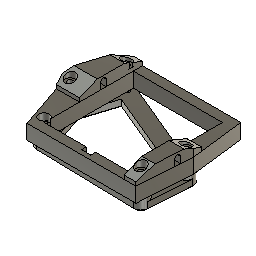
TF4060 rev 5 Heatsink holder (Autodesk Fusion 360 design; units mm, degrees)
Autodesk Fusion 360 part; units mm, degrees
(part 1 of 2)
sketch "68060 socket" plane through (0, 0, 0) normal (0, 0, 1) x (1, 0, 0)
  circle A0 centre (21.59, 21.59) radius 0.4
  circle A1 centre (19.05, 21.59) radius 0.4
  circle A2 centre (16.51, 21.59) radius 0.4
  circle A3 centre (13.97, 21.59) radius 0.4
  circle A4 centre (11.43, 21.59) radius 0.4
  circle A5 centre (8.89, 21.59) radius 0.4
  circle A6 centre (6.35, 21.59) radius 0.4
  circle A7 centre (3.81, 21.59) radius 0.4
  circle A8 centre (1.27, 21.59) radius 0.4
  circle A9 centre (-1.27, 21.59) radius 0.4
  circle A10 centre (-3.81, 21.59) radius 0.4
  circle A11 centre (-6.35, 21.59) radius 0.4
  circle A12 centre (-8.89, 21.59) radius 0.4
  circle A13 centre (-11.43, 21.59) radius 0.4
  circle A14 centre (-13.97, 21.59) radius 0.4
  circle A15 centre (-16.51, 21.59) radius 0.4
  circle A16 centre (-19.05, 21.59) radius 0.4
  circle A17 centre (21.59, 19.05) radius 0.4
  circle A18 centre (21.59, 16.51) radius 0.4
  circle A19 centre (21.59, 13.97) radius 0.4
  circle A20 centre (21.59, 11.43) radius 0.4
  circle A21 centre (21.59, 8.89) radius 0.4
  circle A22 centre (21.59, 6.35) radius 0.4
  circle A23 centre (21.59, 3.81) radius 0.4
  circle A24 centre (21.59, 1.27) radius 0.4
  circle A25 centre (21.59, -1.27) radius 0.4
  circle A26 centre (21.59, -3.81) radius 0.4
  circle A27 centre (21.59, -6.35) radius 0.4
  circle A28 centre (21.59, -8.89) radius 0.4
  circle A29 centre (21.59, -11.43) radius 0.4
  circle A30 centre (21.59, -13.97) radius 0.4
  circle A31 centre (21.59, -16.51) radius 0.4
  circle A32 centre (21.59, -19.05) radius 0.4
  circle A33 centre (21.59, -21.59) radius 0.4
  circle A34 centre (19.05, 19.05) radius 0.4
  circle A35 centre (19.05, 16.51) radius 0.4
  circle A36 centre (19.05, 13.97) radius 0.4
  circle A37 centre (16.51, 19.05) radius 0.4
  circle A38 centre (16.51, 16.51) radius 0.4
  circle A39 centre (16.51, 13.97) radius 0.4
  circle A40 centre (13.97, 19.05) radius 0.4
  circle A41 centre (13.97, 16.51) radius 0.4
  circle A42 centre (13.97, 13.97) radius 0.4
  circle A43 centre (11.43, 19.05) radius 0.4
  circle A44 centre (11.43, 16.51) radius 0.4
  circle A45 centre (11.43, 13.97) radius 0.4
  circle A46 centre (8.89, 19.05) radius 0.4
  circle A47 centre (8.89, 16.51) radius 0.4
  circle A48 centre (8.89, 13.97) radius 0.4
  circle A49 centre (6.35, 19.05) radius 0.4
  circle A50 centre (6.35, 16.51) radius 0.4
  circle A51 centre (6.35, 13.97) radius 0.4
  circle A52 centre (3.81, 19.05) radius 0.4
  circle A53 centre (3.81, 16.51) radius 0.4
  circle A54 centre (3.81, 13.97) radius 0.4
  circle A55 centre (1.27, 19.05) radius 0.4
  circle A56 centre (1.27, 16.51) radius 0.4
  circle A57 centre (1.27, 13.97) radius 0.4
  circle A58 centre (-1.27, 19.05) radius 0.4
  circle A59 centre (-1.27, 16.51) radius 0.4
  circle A60 centre (-1.27, 13.97) radius 0.4
  circle A61 centre (-3.81, 19.05) radius 0.4
  circle A62 centre (-3.81, 16.51) radius 0.4
  circle A63 centre (-3.81, 13.97) radius 0.4
  circle A64 centre (-6.35, 19.05) radius 0.4
  circle A65 centre (-6.35, 16.51) radius 0.4
  circle A66 centre (-6.35, 13.97) radius 0.4
  circle A67 centre (-8.89, 19.05) radius 0.4
  circle A68 centre (-8.89, 16.51) radius 0.4
  circle A69 centre (-8.89, 13.97) radius 0.4
  circle A70 centre (-11.43, 19.05) radius 0.4
  circle A71 centre (-11.43, 16.51) radius 0.4
  circle A72 centre (-11.43, 13.97) radius 0.4
  circle A73 centre (-13.97, 19.05) radius 0.4
  circle A74 centre (-13.97, 16.51) radius 0.4
  circle A75 centre (-13.97, 13.97) radius 0.4
  circle A76 centre (-16.51, 19.05) radius 0.4
  circle A77 centre (-16.51, 16.51) radius 0.4
  circle A78 centre (-16.51, 13.97) radius 0.4
  circle A79 centre (-19.05, 19.05) radius 0.4
  circle A80 centre (-19.05, 16.51) radius 0.4
  circle A81 centre (-19.05, 13.97) radius 0.4
  circle A82 centre (-21.59, 19.05) radius 0.4
  circle A83 centre (-21.59, 16.51) radius 0.4
  circle A84 centre (-21.59, 13.97) radius 0.4
  circle A85 centre (19.05, -21.59) radius 0.4
  circle A86 centre (19.05, -19.05) radius 0.4
  circle A87 centre (19.05, -16.51) radius 0.4
  circle A88 centre (19.05, -13.97) radius 0.4
  circle A89 centre (16.51, -21.59) radius 0.4
  circle A90 centre (16.51, -19.05) radius 0.4
  circle A91 centre (16.51, -16.51) radius 0.4
  circle A92 centre (16.51, -13.97) radius 0.4
  circle A93 centre (13.97, -21.59) radius 0.4
  circle A94 centre (13.97, -19.05) radius 0.4
  circle A95 centre (13.97, -16.51) radius 0.4
  circle A96 centre (13.97, -13.97) radius 0.4
  circle A97 centre (11.43, -21.59) radius 0.4
  circle A98 centre (11.43, -19.05) radius 0.4
  circle A99 centre (11.43, -16.51) radius 0.4
  circle A100 centre (11.43, -13.97) radius 0.4
  circle A101 centre (8.89, -21.59) radius 0.4
  circle A102 centre (8.89, -19.05) radius 0.4
  circle A103 centre (8.89, -16.51) radius 0.4
  circle A104 centre (8.89, -13.97) radius 0.4
  circle A105 centre (6.35, -21.59) radius 0.4
  circle A106 centre (6.35, -19.05) radius 0.4
  circle A107 centre (6.35, -16.51) radius 0.4
  circle A108 centre (6.35, -13.97) radius 0.4
  circle A109 centre (3.81, -21.59) radius 0.4
  circle A110 centre (3.81, -19.05) radius 0.4
  circle A111 centre (3.81, -16.51) radius 0.4
  circle A112 centre (3.81, -13.97) radius 0.4
  circle A113 centre (1.27, -21.59) radius 0.4
  circle A114 centre (1.27, -19.05) radius 0.4
  circle A115 centre (1.27, -16.51) radius 0.4
  circle A116 centre (1.27, -13.97) radius 0.4
  circle A117 centre (-1.27, -21.59) radius 0.4
  circle A118 centre (-1.27, -19.05) radius 0.4
  circle A119 centre (-1.27, -16.51) radius 0.4
  circle A120 centre (-1.27, -13.97) radius 0.4
  circle A121 centre (-3.81, -21.59) radius 0.4
  circle A122 centre (-3.81, -19.05) radius 0.4
  circle A123 centre (-3.81, -16.51) radius 0.4
  circle A124 centre (-3.81, -13.97) radius 0.4
  circle A125 centre (-6.35, -21.59) radius 0.4
  circle A126 centre (-6.35, -19.05) radius 0.4
  circle A127 centre (-6.35, -16.51) radius 0.4
  circle A128 centre (-6.35, -13.97) radius 0.4
  circle A129 centre (-8.89, -21.59) radius 0.4
  circle A130 centre (-8.89, -19.05) radius 0.4
  circle A131 centre (-8.89, -16.51) radius 0.4
  circle A132 centre (-8.89, -13.97) radius 0.4
  circle A133 centre (-11.43, -21.59) radius 0.4
  circle A134 centre (-11.43, -19.05) radius 0.4
  circle A135 centre (-11.43, -16.51) radius 0.4
  circle A136 centre (-11.43, -13.97) radius 0.4
  circle A137 centre (-13.97, -21.59) radius 0.4
  circle A138 centre (-13.97, -19.05) radius 0.4
  circle A139 centre (-13.97, -16.51) radius 0.4
  circle A140 centre (-13.97, -13.97) radius 0.4
  circle A141 centre (-16.51, -21.59) radius 0.4
  circle A142 centre (-16.51, -19.05) radius 0.4
  circle A143 centre (-16.51, -16.51) radius 0.4
  circle A144 centre (-16.51, -13.97) radius 0.4
  circle A145 centre (-19.05, -21.59) radius 0.4
  circle A146 centre (-19.05, -19.05) radius 0.4
  circle A147 centre (-19.05, -16.51) radius 0.4
  circle A148 centre (-19.05, -13.97) radius 0.4
  circle A149 centre (-21.59, -21.59) radius 0.4
  circle A150 centre (-21.59, -19.05) radius 0.4
  circle A151 centre (-21.59, -16.51) radius 0.4
  circle A152 centre (-21.59, -13.97) radius 0.4
  circle A153 centre (19.05, -11.43) radius 0.4
  circle A154 centre (16.51, -11.43) radius 0.4
  circle A155 centre (13.97, -11.43) radius 0.4
  circle A156 centre (-13.97, -11.43) radius 0.4
  circle A157 centre (-16.51, -11.43) radius 0.4
  circle A158 centre (-19.05, -11.43) radius 0.4
  circle A159 centre (-21.59, -11.43) radius 0.4
  circle A160 centre (19.05, -8.89) radius 0.4
  circle A161 centre (16.51, -8.89) radius 0.4
  circle A162 centre (13.97, -8.89) radius 0.4
  circle A163 centre (-13.97, -8.89) radius 0.4
  circle A164 centre (-16.51, -8.89) radius 0.4
  circle A165 centre (-19.05, -8.89) radius 0.4
  circle A166 centre (-21.59, -8.89) radius 0.4
  circle A167 centre (19.05, -6.35) radius 0.4
  circle A168 centre (16.51, -6.35) radius 0.4
  circle A169 centre (13.97, -6.35) radius 0.4
  circle A170 centre (-13.97, -6.35) radius 0.4
  circle A171 centre (-16.51, -6.35) radius 0.4
  circle A172 centre (-19.05, -6.35) radius 0.4
  circle A173 centre (-21.59, -6.35) radius 0.4
  circle A174 centre (19.05, -3.81) radius 0.4
  circle A175 centre (16.51, -3.81) radius 0.4
  circle A176 centre (13.97, -3.81) radius 0.4
  circle A177 centre (-13.97, -3.81) radius 0.4
  circle A178 centre (-16.51, -3.81) radius 0.4
  circle A179 centre (-19.05, -3.81) radius 0.4
  circle A180 centre (-21.59, -3.81) radius 0.4
  circle A181 centre (19.05, -1.27) radius 0.4
  circle A182 centre (16.51, -1.27) radius 0.4
  circle A183 centre (13.97, -1.27) radius 0.4
  circle A184 centre (-13.97, -1.27) radius 0.4
  circle A185 centre (-16.51, -1.27) radius 0.4
  circle A186 centre (-19.05, -1.27) radius 0.4
  circle A187 centre (-21.59, -1.27) radius 0.4
  circle A188 centre (19.05, 1.27) radius 0.4
  circle A189 centre (16.51, 1.27) radius 0.4
  circle A190 centre (13.97, 1.27) radius 0.4
  circle A191 centre (-13.97, 1.27) radius 0.4
  circle A192 centre (-16.51, 1.27) radius 0.4
  circle A193 centre (-19.05, 1.27) radius 0.4
  circle A194 centre (-21.59, 1.27) radius 0.4
  circle A195 centre (19.05, 3.81) radius 0.4
  circle A196 centre (16.51, 3.81) radius 0.4
  circle A197 centre (13.97, 3.81) radius 0.4
  circle A198 centre (-13.97, 3.81) radius 0.4
  circle A199 centre (-16.51, 3.81) radius 0.4
  circle A200 centre (-19.05, 3.81) radius 0.4
  circle A201 centre (-21.59, 3.81) radius 0.4
  circle A202 centre (19.05, 6.35) radius 0.4
  circle A203 centre (16.51, 6.35) radius 0.4
  circle A204 centre (13.97, 6.35) radius 0.4
  circle A205 centre (-13.97, 6.35) radius 0.4
  circle A206 centre (-16.51, 6.35) radius 0.4
  circle A207 centre (-19.05, 6.35) radius 0.4
  circle A208 centre (-21.59, 6.35) radius 0.4
  circle A209 centre (19.05, 8.89) radius 0.4
  circle A210 centre (16.51, 8.89) radius 0.4
  circle A211 centre (13.97, 8.89) radius 0.4
  circle A212 centre (-13.97, 8.89) radius 0.4
  circle A213 centre (-16.51, 8.89) radius 0.4
  circle A214 centre (-19.05, 8.89) radius 0.4
  circle A215 centre (-21.59, 8.89) radius 0.4
  circle A216 centre (19.05, 11.43) radius 0.4
  circle A217 centre (16.51, 11.43) radius 0.4
  circle A218 centre (13.97, 11.43) radius 0.4
  circle A219 centre (-13.97, 11.43) radius 0.4
  circle A220 centre (-16.51, 11.43) radius 0.4
  circle A221 centre (-19.05, 11.43) radius 0.4
  circle A222 centre (-21.59, 11.43) radius 0.4
  dimension "d1" = 0.8
  dimension "d2" = 21.59
  dimension "d3" = 21.59
  dimension "d6" = -2.54
  dimension "d7" = 0
  dimension "d10" = 0
  dimension "d11" = -2.54
  dimension "d14" = -2.54
  dimension "d15" = 0
  dimension "d18" = -2.54
  dimension "d19" = 0
  dimension "d22" = 0
  dimension "d23" = 2.54
  measures "d1" diameter of A0
  measures "d2" horizontal distance of origin A0.centre
  measures "d3" vertical distance of origin A0.centre
sketch "Header pins" plane through (0, 0, 0) normal (0, 0, 1) x (1, 0, 0)
  circle A0 centre (-0.0505, -25.4404) radius 0.508
  circle A1 centre (2.4895, -25.4404) radius 0.508
  circle A2 centre (-9.1793, -28.3555) radius 0.508
  circle A3 centre (-11.7193, -28.3555) radius 0.508
  circle A4 centre (-14.2593, -28.3555) radius 0.508
  circle A5 centre (-26.6083, 15.9484) radius 0.508
  circle A6 centre (-26.6083, 18.4884) radius 0.508
  circle A7 centre (-29.1428, 18.4884) radius 0.508
  circle A8 centre (-31.6883, 18.4884) radius 0.508
  circle A9 centre (-29.1428, 15.9484) radius 0.508
  circle A10 centre (-31.6883, 15.9484) radius 0.508
  dimension "d24" = 1.016
  dimension "d25" = 0.0505
  dimension "d26" = 25.4404
  dimension "d27" = 1.016
  dimension "d28" = 2.4895
  dimension "d29" = 9.1793
  dimension "d30" = 11.7193
  dimension "d31" = 14.2593
  dimension "d32" = 28.3555
  dimension "d33" = 1.016
  dimension "d34" = 1.016
  dimension "d35" = 1.016
  dimension "d36" = 15.9484
  dimension "d37" = 18.4884
  dimension "d38" = 26.6083
  dimension "d39" = 29.1428
  dimension "d40" = 31.6883
  dimension "d41" = 1.016
  dimension "d42" = 1.016
  dimension "d43" = 1.016
  dimension "d44" = 1.016
  dimension "d45" = 1.016
  dimension "d46" = 1.016
  constraint horizontal A0.centre A1.centre
  constraint horizontal A3.centre A4.centre
  constraint horizontal A2.centre A3.centre
  constraint horizontal A6.centre A7.centre
  constraint horizontal A7.centre A8.centre
  constraint vertical A5.centre A6.centre
  constraint vertical A7.centre A9.centre
  constraint vertical A8.centre A10.centre
  constraint horizontal A5.centre A9.centre
  constraint horizontal A9.centre A10.centre
  measures "d24" diameter of A0
  measures "d25" horizontal distance of A0.centre origin
  measures "d26" vertical distance of A0.centre origin
  measures "d27" diameter of A1
  measures "d28" horizontal distance of origin A1.centre
  measures "d29" horizontal distance of origin A2.centre
  measures "d30" horizontal distance of origin A3.centre
  measures "d31" horizontal distance of origin A4.centre
  measures "d32" vertical distance of origin A4.centre
  measures "d33" diameter of A2
  measures "d34" diameter of A3
  measures "d35" diameter of A4
  measures "d36" vertical distance of origin A5.centre
  measures "d37" vertical distance of origin A6.centre
  measures "d38" horizontal distance of origin A6.centre
  measures "d39" horizontal distance of origin A7.centre
  measures "d40" horizontal distance of origin A8.centre
  measures "d41" diameter of A6
  measures "d42" diameter of A7
  measures "d43" diameter of A8
  measures "d44" diameter of A5
  measures "d45" diameter of A9
  measures "d46" diameter of A10
sketch "Mounting holes" plane through (0, 0, 0) normal (0, 0, 1) x (1, 0, 0)
  circle A0 centre (-34.0203, -0.0351) radius 1.27
  line L0 (-50, 0) -> (50, 0) construction
  line L1 (0, 50) -> (0, -50) construction
  circle A1 centre (-26.7388, -21.5341) radius 1.27
  circle A2 centre (-26.7388, 23.0505) radius 1.27
  circle A3 centre (26.9591, -22.8364) radius 1.27
  circle A4 centre (28.498, 0) radius 1.27
  circle A5 centre (-19.05, 21.59) radius 0.4 construction
  circle A6 centre (-16.51, 21.59) radius 0.4 construction
  circle A7 centre (-13.97, 21.59) radius 0.4 construction
  circle A8 centre (-11.43, 21.59) radius 0.4 construction
  circle A9 centre (-8.89, 21.59) radius 0.4 construction
  circle A10 centre (-6.35, 21.59) radius 0.4 construction
  circle A11 centre (-3.81, 21.59) radius 0.4 construction
  circle A12 centre (-1.27, 21.59) radius 0.4 construction
  circle A13 centre (1.27, 21.59) radius 0.4 construction
  circle A14 centre (3.81, 21.59) radius 0.4 construction
  circle A15 centre (6.35, 21.59) radius 0.4 construction
  circle A16 centre (8.89, 21.59) radius 0.4 construction
  circle A17 centre (11.43, 21.59) radius 0.4 construction
  circle A18 centre (13.97, 21.59) radius 0.4 construction
  circle A19 centre (16.51, 21.59) radius 0.4 construction
  circle A20 centre (19.05, 21.59) radius 0.4 construction
  circle A21 centre (21.59, 21.59) radius 0.4 construction
  circle A22 centre (21.59, 19.05) radius 0.4 construction
  circle A23 centre (19.05, 19.05) radius 0.4 construction
  circle A24 centre (16.51, 19.05) radius 0.4 construction
  circle A25 centre (13.97, 19.05) radius 0.4 construction
  circle A26 centre (11.43, 19.05) radius 0.4 construction
  circle A27 centre (8.89, 19.05) radius 0.4 construction
  circle A28 centre (6.35, 19.05) radius 0.4 construction
  circle A29 centre (3.81, 19.05) radius 0.4 construction
  circle A30 centre (1.27, 19.05) radius 0.4 construction
  circle A31 centre (-1.27, 19.05) radius 0.4 construction
  circle A32 centre (-3.81, 19.05) radius 0.4 construction
  circle A33 centre (-6.35, 19.05) radius 0.4 construction
  circle A34 centre (-8.89, 19.05) radius 0.4 construction
  circle A35 centre (-11.43, 19.05) radius 0.4 construction
  circle A36 centre (-13.97, 19.05) radius 0.4 construction
  circle A37 centre (-16.51, 19.05) radius 0.4 construction
  circle A38 centre (-19.05, 19.05) radius 0.4 construction
  circle A39 centre (-21.59, 19.05) radius 0.4 construction
  circle A40 centre (-21.59, 16.51) radius 0.4 construction
  circle A41 centre (-19.05, 16.51) radius 0.4 construction
  circle A42 centre (-16.51, 16.51) radius 0.4 construction
  circle A43 centre (-13.97, 16.51) radius 0.4 construction
  circle A44 centre (-11.43, 16.51) radius 0.4 construction
  circle A45 centre (-8.89, 16.51) radius 0.4 construction
  circle A46 centre (-6.35, 16.51) radius 0.4 construction
  circle A47 centre (-3.81, 16.51) radius 0.4 construction
  circle A48 centre (-1.27, 16.51) radius 0.4 construction
  circle A49 centre (1.27, 16.51) radius 0.4 construction
  circle A50 centre (3.81, 16.51) radius 0.4 construction
  circle A51 centre (6.35, 16.51) radius 0.4 construction
  circle A52 centre (8.89, 16.51) radius 0.4 construction
  circle A53 centre (11.43, 16.51) radius 0.4 construction
  circle A54 centre (13.97, 16.51) radius 0.4 construction
  circle A55 centre (16.51, 16.51) radius 0.4 construction
  circle A56 centre (19.05, 16.51) radius 0.4 construction
  circle A57 centre (21.59, 16.51) radius 0.4 construction
  circle A58 centre (21.59, 13.97) radius 0.4 construction
  circle A59 centre (19.05, 13.97) radius 0.4 construction
  circle A60 centre (16.51, 13.97) radius 0.4 construction
  circle A61 centre (13.97, 13.97) radius 0.4 construction
  circle A62 centre (11.43, 13.97) radius 0.4 construction
  circle A63 centre (8.89, 13.97) radius 0.4 construction
  circle A64 centre (6.35, 13.97) radius 0.4 construction
  circle A65 centre (3.81, 13.97) radius 0.4 construction
  circle A66 centre (1.27, 13.97) radius 0.4 construction
  circle A67 centre (-1.27, 13.97) radius 0.4 construction
  circle A68 centre (-3.81, 13.97) radius 0.4 construction
  circle A69 centre (-6.35, 13.97) radius 0.4 construction
  circle A70 centre (-8.89, 13.97) radius 0.4 construction
  circle A71 centre (-11.43, 13.97) radius 0.4 construction
  circle A72 centre (-13.97, 13.97) radius 0.4 construction
  circle A73 centre (-16.51, 13.97) radius 0.4 construction
  circle A74 centre (-19.05, 13.97) radius 0.4 construction
  circle A75 centre (-21.59, 13.97) radius 0.4 construction
  circle A76 centre (-21.59, 11.43) radius 0.4 construction
  circle A77 centre (-19.05, 11.43) radius 0.4 construction
  circle A78 centre (-16.51, 11.43) radius 0.4 construction
  circle A79 centre (-13.97, 11.43) radius 0.4 construction
  circle A80 centre (13.97, 11.43) radius 0.4 construction
  circle A81 centre (16.51, 11.43) radius 0.4 construction
  circle A82 centre (19.05, 11.43) radius 0.4 construction
  circle A83 centre (21.59, 11.43) radius 0.4 construction
  circle A84 centre (21.59, 8.89) radius 0.4 construction
  circle A85 centre (19.05, 8.89) radius 0.4 construction
  circle A86 centre (16.51, 8.89) radius 0.4 construction
  circle A87 centre (13.97, 8.89) radius 0.4 construction
  circle A88 centre (13.97, 6.35) radius 0.4 construction
  circle A89 centre (16.51, 6.35) radius 0.4 construction
  circle A90 centre (19.05, 6.35) radius 0.4 construction
  circle A91 centre (21.59, 6.35) radius 0.4 construction
  circle A92 centre (21.59, 3.81) radius 0.4 construction
  circle A93 centre (19.05, 3.81) radius 0.4 construction
  circle A94 centre (16.51, 3.81) radius 0.4 construction
  circle A95 centre (13.97, 3.81) radius 0.4 construction
  circle A96 centre (13.97, 1.27) radius 0.4 construction
  circle A97 centre (16.51, 1.27) radius 0.4 construction
  circle A98 centre (19.05, 1.27) radius 0.4 construction
  circle A99 centre (21.59, 1.27) radius 0.4 construction
  circle A100 centre (-13.97, 8.89) radius 0.4 construction
  circle A101 centre (-16.51, 8.89) radius 0.4 construction
  circle A102 centre (-19.05, 8.89) radius 0.4 construction
  circle A103 centre (-21.59, 8.89) radius 0.4 construction
  circle A104 centre (-21.59, 6.35) radius 0.4 construction
  circle A105 centre (-19.05, 6.35) radius 0.4 construction
  circle A106 centre (-16.51, 6.35) radius 0.4 construction
  circle A107 centre (-13.97, 6.35) radius 0.4 construction
  circle A108 centre (-13.97, 3.81) radius 0.4 construction
  circle A109 centre (-16.51, 3.81) radius 0.4 construction
  circle A110 centre (-19.05, 3.81) radius 0.4 construction
  circle A111 centre (-21.59, 3.81) radius 0.4 construction
  circle A112 centre (-21.59, 1.27) radius 0.4 construction
  circle A113 centre (-19.05, 1.27) radius 0.4 construction
  circle A114 centre (-16.51, 1.27) radius 0.4 construction
  circle A115 centre (-13.97, 1.27) radius 0.4 construction
  circle A116 centre (21.59, -1.27) radius 0.4 construction
  circle A117 centre (19.05, -1.27) radius 0.4 construction
  circle A118 centre (16.51, -1.27) radius 0.4 construction
  circle A119 centre (13.97, -1.27) radius 0.4 construction
  circle A120 centre (-13.97, -1.27) radius 0.4 construction
  circle A121 centre (-16.51, -1.27) radius 0.4 construction
  circle A122 centre (-19.05, -1.27) radius 0.4 construction
  circle A123 centre (-21.59, -1.27) radius 0.4 construction
  circle A124 centre (-21.59, -3.81) radius 0.4 construction
  circle A125 centre (-19.05, -3.81) radius 0.4 construction
  circle A126 centre (-16.51, -3.81) radius 0.4 construction
  circle A127 centre (-13.97, -3.81) radius 0.4 construction
  circle A128 centre (-13.97, -6.35) radius 0.4 construction
  circle A129 centre (-16.51, -6.35) radius 0.4 construction
  circle A130 centre (-19.05, -6.35) radius 0.4 construction
  circle A131 centre (-21.59, -6.35) radius 0.4 construction
  circle A132 centre (-21.59, -8.89) radius 0.4 construction
  circle A133 centre (-19.05, -8.89) radius 0.4 construction
  circle A134 centre (-16.51, -8.89) radius 0.4 construction
  circle A135 centre (-13.97, -8.89) radius 0.4 construction
  circle A136 centre (-13.97, -11.43) radius 0.4 construction
  circle A137 centre (-16.51, -11.43) radius 0.4 construction
  circle A138 centre (-19.05, -11.43) radius 0.4 construction
  circle A139 centre (-21.59, -11.43) radius 0.4 construction
  circle A140 centre (13.97, -3.81) radius 0.4 construction
  circle A141 centre (21.59, -3.81) radius 0.4 construction
  circle A142 centre (19.05, -3.81) radius 0.4 construction
  circle A143 centre (16.51, -3.81) radius 0.4 construction
  circle A144 centre (21.59, -6.35) radius 0.4 construction
  circle A145 centre (19.05, -6.35) radius 0.4 construction
  circle A146 centre (16.51, -6.35) radius 0.4 construction
  circle A147 centre (13.97, -6.35) radius 0.4 construction
  circle A148 centre (21.59, -8.89) radius 0.4 construction
  circle A149 centre (19.05, -8.89) radius 0.4 construction
  circle A150 centre (16.51, -8.89) radius 0.4 construction
  circle A151 centre (13.97, -8.89) radius 0.4 construction
  circle A152 centre (21.59, -11.43) radius 0.4 construction
  circle A153 centre (19.05, -11.43) radius 0.4 construction
  circle A154 centre (16.51, -11.43) radius 0.4 construction
  circle A155 centre (13.97, -11.43) radius 0.4 construction
  circle A156 centre (21.59, -13.97) radius 0.4 construction
  circle A157 centre (19.05, -13.97) radius 0.4 construction
  circle A158 centre (16.51, -13.97) radius 0.4 construction
  circle A159 centre (13.97, -13.97) radius 0.4 construction
  circle A160 centre (11.43, -13.97) radius 0.4 construction
  circle A161 centre (8.89, -13.97) radius 0.4 construction
  circle A162 centre (6.35, -13.97) radius 0.4 construction
  circle A163 centre (3.81, -13.97) radius 0.4 construction
  circle A164 centre (1.27, -13.97) radius 0.4 construction
  circle A165 centre (-1.27, -13.97) radius 0.4 construction
  circle A166 centre (-3.81, -13.97) radius 0.4 construction
  circle A167 centre (-6.35, -13.97) radius 0.4 construction
  circle A168 centre (-8.89, -13.97) radius 0.4 construction
  circle A169 centre (-11.43, -13.97) radius 0.4 construction
  circle A170 centre (-13.97, -13.97) radius 0.4 construction
  circle A171 centre (-16.51, -13.97) radius 0.4 construction
  circle A172 centre (-19.05, -13.97) radius 0.4 construction
  circle A173 centre (-21.59, -13.97) radius 0.4 construction
  circle A174 centre (21.59, -16.51) radius 0.4 construction
  circle A175 centre (19.05, -16.51) radius 0.4 construction
  circle A176 centre (16.51, -16.51) radius 0.4 construction
  circle A177 centre (13.97, -16.51) radius 0.4 construction
  circle A178 centre (11.43, -16.51) radius 0.4 construction
  circle A179 centre (8.89, -16.51) radius 0.4 construction
  circle A180 centre (6.35, -16.51) radius 0.4 construction
  circle A181 centre (3.81, -16.51) radius 0.4 construction
  circle A182 centre (-1.27, -16.51) radius 0.4 construction
  circle A183 centre (1.27, -16.51) radius 0.4 construction
  circle A184 centre (-3.81, -16.51) radius 0.4 construction
  circle A185 centre (-6.35, -16.51) radius 0.4 construction
  circle A186 centre (-8.89, -16.51) radius 0.4 construction
  circle A187 centre (-11.43, -16.51) radius 0.4 construction
  circle A188 centre (-13.97, -16.51) radius 0.4 construction
  circle A189 centre (-16.51, -16.51) radius 0.4 construction
  circle A190 centre (-19.05, -16.51) radius 0.4 construction
  circle A191 centre (-21.59, -16.51) radius 0.4 construction
  circle A192 centre (21.59, -19.05) radius 0.4 construction
  circle A193 centre (19.05, -19.05) radius 0.4 construction
  circle A194 centre (16.51, -19.05) radius 0.4 construction
  circle A195 centre (13.97, -19.05) radius 0.4 construction
  circle A196 centre (11.43, -19.05) radius 0.4 construction
  circle A197 centre (8.89, -19.05) radius 0.4 construction
  circle A198 centre (6.35, -19.05) radius 0.4 construction
  circle A199 centre (3.81, -19.05) radius 0.4 construction
  circle A200 centre (1.27, -19.05) radius 0.4 construction
  circle A201 centre (-1.27, -19.05) radius 0.4 construction
  circle A202 centre (-3.81, -19.05) radius 0.4 construction
  circle A203 centre (-6.35, -19.05) radius 0.4 construction
  circle A204 centre (-8.89, -19.05) radius 0.4 construction
  circle A205 centre (-11.43, -19.05) radius 0.4 construction
  circle A206 centre (-13.97, -19.05) radius 0.4 construction
  circle A207 centre (-16.51, -19.05) radius 0.4 construction
  circle A208 centre (-19.05, -19.05) radius 0.4 construction
  circle A209 centre (-21.59, -19.05) radius 0.4 construction
  circle A210 centre (21.59, -21.59) radius 0.4 construction
  circle A211 centre (19.05, -21.59) radius 0.4 construction
  circle A212 centre (16.51, -21.59) radius 0.4 construction
  circle A213 centre (13.97, -21.59) radius 0.4 construction
  circle A214 centre (11.43, -21.59) radius 0.4 construction
  circle A215 centre (8.89, -21.59) radius 0.4 construction
  circle A216 centre (6.35, -21.59) radius 0.4 construction
  circle A217 centre (3.81, -21.59) radius 0.4 construction
  circle A218 centre (1.27, -21.59) radius 0.4 construction
  circle A219 centre (-1.27, -21.59) radius 0.4 construction
  circle A220 centre (-3.81, -21.59) radius 0.4 construction
  circle A221 centre (-6.35, -21.59) radius 0.4 construction
  circle A222 centre (-8.89, -21.59) radius 0.4 construction
  circle A223 centre (-11.43, -21.59) radius 0.4 construction
  circle A224 centre (-13.97, -21.59) radius 0.4 construction
  circle A225 centre (-16.51, -21.59) radius 0.4 construction
  circle A226 centre (-19.05, -21.59) radius 0.4 construction
  circle A227 centre (-21.59, -21.59) radius 0.4 construction
  circle A228 centre (2.4895, -25.4404) radius 0.508 construction
  circle A229 centre (-0.0505, -25.4404) radius 0.508 construction
  circle A230 centre (-9.1793, -28.3555) radius 0.508 construction
  circle A231 centre (-11.7193, -28.3555) radius 0.508 construction
  circle A232 centre (-14.2593, -28.3555) radius 0.508 construction
  circle A233 centre (-26.6083, 15.9484) radius 0.508 construction
  circle A234 centre (-26.6083, 18.4884) radius 0.508 construction
  circle A235 centre (-29.1428, 18.4884) radius 0.508 construction
  circle A236 centre (-29.1428, 15.9484) radius 0.508 construction
  circle A237 centre (-31.6883, 18.4884) radius 0.508 construction
  circle A238 centre (-31.6883, 15.9484) radius 0.508 construction
  line L2 (-23.6, 23.6) -> (23.6, 23.6) construction
  line L3 (23.6, 23.6) -> (23.6, -23.6) construction
  line L4 (23.6, -23.6) -> (-23.6, -23.6) construction
  line L5 (-23.6, -23.6) -> (-23.6, 23.6) construction
  dimension "d48" = 34.0203
  dimension "d49" = 0.0351
  dimension "d50" = 26.7388
  dimension "d51" = 21.5341
  dimension "d52" = 26.7388
  dimension "d53" = 23.0505
  dimension "d54" = 26.9591
  dimension "d55" = 22.8364
  dimension "d56" = 28.498
  dimension "d57" = 2.54
  dimension "d58" = 2.54
  dimension "d59" = 2.54
  dimension "d60" = 2.54
  dimension "d61" = 2.54
  dimension "d62" = 47.2
  dimension "d63" = 47.2
  dimension "d64" = 23.6
  dimension "d65" = 23.6
  constraint horizontal L0
  constraint vertical L1
  constraint coincident L0 A4.centre
  constraint horizontal L2
  constraint vertical L3
  constraint horizontal L4
  constraint vertical L5
  measures "d48" distance of A0.centre L1
  measures "d49" distance of A0.centre L0
  measures "d50" distance of L1 A1.centre
  measures "d51" distance of L0 A1.centre
  measures "d52" distance of L1 A2.centre
  measures "d53" distance of L0 A2.centre
  measures "d54" distance of L1 A3.centre
  measures "d55" distance of L0 A3.centre
  measures "d56" distance of L1 A4.centre
  measures "d57" diameter of A4
  measures "d58" diameter of A3
  measures "d59" diameter of A1
  measures "d60" diameter of A0
  measures "d61" diameter of A2
  measures "d62" distance of L2.start L2.end
  measures "d63" distance of L2.end L3.end
  measures "d64" distance of L1 L3
  measures "d65" distance of L0 L2
sketch "Bottom frame" plane through (0, 0, 0) normal (0, 0, 1) x (1, 0, 0) in component "Bottom frame"
  circle A0 centre (-26.7388, 23.0505) radius 1.5
  circle A1 centre (-34.0203, -0.0351) radius 1.5
  circle A2 centre (-26.7388, -21.5341) radius 1.5
  circle A3 centre (26.9591, -22.8364) radius 1.5
  circle A4 centre (28.498, 0) radius 1.5
  circle A5 centre (-26.7388, 23.0505) radius 4
  circle A6 centre (-34.0203, -0.0351) radius 4
  circle A7 centre (-26.7388, -21.5341) radius 4
  circle A8 centre (26.9591, -22.8364) radius 4
  circle A9 centre (28.498, 0) radius 4
  line L0 (-24.2405, 17.6736) -> (-29.812, 0.0092)
  line L1 (32.489, -0.269) -> (30.95, -23.1053)
  line L2 (26.8621, -26.8352) -> (-26.8358, -25.5329)
  line L3 (-30.5274, -22.8173) -> (-37.8089, -1.3182)
  line L4 (-37.835, 1.1682) -> (-30.5536, 24.2537)
  line L5 (-30.2316, 1.2481) -> (-23.847, -17.6031)
  line L6 (24.3145, -2.5885) -> (23.2257, -18.7447)
  line L7 (-23.847, -17.6031) -> (23.2257, -18.7447)
  line L8 (-24.2405, 17.6736) -> (24.3145, -2.5885)
  line L9 (30.0385, 3.6915) -> (-25.1984, 26.742)
  line L10 (-26.7388, 27.0505) -> (-26.7388, 19.0505)
  line L11 (-34.0203, -0.0351) -> (-30.0203, -0.0351)
  line L12 (-34.0203, -0.0351) -> (-34.0203, -4.0351)
  point P0 (-26.7388, 23.0505)
  point P1 (-34.0203, -0.0351)
  point P2 (-26.7388, -21.5341)
  point P3 (26.9591, -22.8364)
  point P4 (28.498, 0)
  dimension "d66" = 3
  dimension "d67" = 3
  dimension "d68" = 3
  dimension "d69" = 3
  dimension "d70" = 3
  dimension "d71" = 8
  dimension "d72" = 8
  dimension "d73" = 8
  dimension "d74" = 8
  dimension "d75" = 8
  constraint coincident P0 A0.centre
  constraint coincident P1 A1.centre
  constraint coincident P2 A2.centre
  constraint coincident P3 A3.centre
  constraint coincident P4 A4.centre
  constraint concentric A0 A5
  constraint concentric A4 A9
  constraint tangent A5 L0
  constraint tangent A6 L0
  constraint tangent A7 L2
  constraint tangent A7 L3
  constraint tangent A6 L3
  constraint tangent A6 L4
  constraint tangent A5 L4
  constraint tangent A9 L1
  constraint tangent A8 L1
  constraint tangent A8 L2
  constraint tangent A6 L5
  constraint tangent A7 L5
  constraint tangent A7 L7
  constraint tangent A8 L7
  constraint tangent A8 L6
  constraint tangent A9 L6
  constraint coincident A6 L5.start
  constraint coincident A9 L1.start
  constraint coincident A5 L4.end
  constraint coincident A6 L4.start
  constraint coincident A6 L3.end
  constraint coincident A7 L3.start
  constraint coincident A7 L2.end
  constraint coincident A8 L2.start
  constraint coincident A8 L1.end
  constraint tangent A5 L9
  constraint tangent A9 L9
  constraint tangent A9 L8
  constraint tangent A5 L8
  constraint coincident A9 L9.start
  constraint coincident A5 L9.end
  constraint coincident A5 L10.start
  constraint coincident A5 L10.end
  constraint vertical L10
  constraint midpoint P0 L10
  constraint coincident A6 L11.end
  constraint horizontal L11
  constraint coincident A6 L12.end
  constraint perpendicular L11 L12
  measures "d66" diameter of A0
  measures "d67" diameter of A1
  measures "d68" diameter of A2
  measures "d69" diameter of A4
  measures "d70" diameter of A3
  measures "d71" diameter of A5
  measures "d72" diameter of A6
  measures "d73" diameter of A7
  measures "d74" diameter of A9
  measures "d75" diameter of A8
extrude "Extrude1" add sketch "Bottom frame" along normal blind 2 contours A0 A5 L10 | A9 | A1 A6 L11 L12 | A8 | A7 picked at (-29.8139, 23.7768) picked at (-36.9614, 1.1182) makes body 1 at (-22.7587, -21.1358, 1.3333) makes body 2 at (-33.824, 3.9601, 0.6667) makes body 3 at (25.6851, -19.0447, 0.6667) makes body 4 at (-29.1541, 26.239, 1.3333) makes body 5 at (28.3983, -3.9988, 0.6667) in component "Bottom frame"
extrude "Extrude2" add sketch "Bottom frame" against normal blind 4 contours A0 A5 L10 | A0 A5 L10 | A5 A6 A7 A8 A9 L1 L2 L3 L4 L9 | A9 | A1 A6 L11 L12 | A8 | A1 A6 L11 L12 | A7 bodies 1 2 3 4 5 in component "Bottom frame"
sketch "Nut countersink" plane through (0, 0, -4) normal (0, 0, -1) x (1, 0, 0) in component "Bottom frame"
  circle A0 centre (28.498, 0) radius 1.5
  circle A1 centre (-26.7388, 21.5341) radius 1.5
  circle A2 centre (26.9591, 22.8364) radius 1.5
  circle A3 centre (-26.7388, -23.0505) radius 1.5
  circle A4 centre (-34.0203, 0.0351) radius 1.5
  line L0 (-29.812, -0.0092) -> (-23.847, 17.6031)
  line L1 (-23.847, 17.6031) -> (23.2257, 18.7447)
  line L2 (23.2257, 18.7447) -> (24.3145, 2.5885)
  line L3 (24.3145, 2.5885) -> (-24.2405, -17.6736)
  line L4 (-24.2405, -17.6736) -> (-29.812, -0.0092)
  arc A5 (30.0385, -3.6915) -> (32.489, 0.269) centre (28.498, 0) ccw
  line L5 (32.489, 0.269) -> (30.95, 23.1053)
  arc A6 (30.95, 23.1053) -> (26.8621, 26.8352) centre (26.9591, 22.8364) ccw
  line L6 (26.8621, 26.8352) -> (-26.8358, 25.5329)
  arc A7 (-26.8358, 25.5329) -> (-30.5274, 22.8173) centre (-26.7388, 21.5341) ccw
  line L7 (-30.5274, 22.8173) -> (-37.8089, 1.3182)
  arc A8 (-37.8089, 1.3182) -> (-37.835, -1.1682) centre (-34.0203, 0.0351) ccw
  line L8 (-37.835, -1.1682) -> (-30.5536, -24.2537)
  arc A9 (-30.5536, -24.2537) -> (-25.1984, -26.742) centre (-26.7388, -23.0505) ccw
  line L9 (-25.1984, -26.742) -> (30.0385, -3.6915)
  line L10 (25.948, -1.4722) -> (28.498, -2.9445)
  line L11 (28.498, -2.9445) -> (31.048, -1.4722)
  line L12 (31.048, -1.4722) -> (31.048, 1.4722)
  line L13 (31.048, 1.4722) -> (28.498, 2.9445)
  line L14 (28.498, 2.9445) -> (25.948, 1.4722)
  line L15 (25.948, 1.4722) -> (25.948, -1.4722)
  line L16 (24.4091, 21.3641) -> (26.9591, 19.8919)
  line L17 (26.9591, 19.8919) -> (29.5091, 21.3641)
  line L18 (29.5091, 21.3641) -> (29.5091, 24.3086)
  line L19 (29.5091, 24.3086) -> (26.9591, 25.7809)
  line L20 (26.9591, 25.7809) -> (24.4091, 24.3086)
  line L21 (24.4091, 24.3086) -> (24.4091, 21.3641)
  line L22 (-29.2888, -24.5227) -> (-26.7388, -25.995)
  line L23 (-26.7388, -25.995) -> (-24.1888, -24.5227)
  line L24 (-24.1888, -24.5227) -> (-24.1888, -21.5783)
  line L25 (-24.1888, -21.5783) -> (-26.7388, -20.106)
  line L26 (-26.7388, -20.106) -> (-29.2888, -21.5783)
  line L27 (-29.2888, -21.5783) -> (-29.2888, -24.5227)
  line L28 (-36.5703, -1.4372) -> (-34.0203, -2.9094)
  line L29 (-34.0203, -2.9094) -> (-31.4703, -1.4372)
  line L30 (-31.4703, -1.4372) -> (-31.4703, 1.5073)
  line L31 (-31.4703, 1.5073) -> (-34.0203, 2.9795)
  line L32 (-34.0203, 2.9795) -> (-36.5703, 1.5073)
  line L33 (-36.5703, 1.5073) -> (-36.5703, -1.4372)
  line L34 (-29.2888, 20.0619) -> (-26.7388, 18.5896)
  line L35 (-26.7388, 18.5896) -> (-24.1888, 20.0619)
  line L36 (-24.1888, 20.0619) -> (-24.1888, 23.0064)
  line L37 (-24.1888, 23.0064) -> (-26.7388, 24.4786)
  line L38 (-26.7388, 24.4786) -> (-29.2888, 23.0064)
  line L39 (-29.2888, 23.0064) -> (-29.2888, 20.0619)
  point P0 (28.498, 0)
  point P1 (26.9591, 22.8364)
  point P2 (-26.7388, -23.0505)
  point P3 (-26.7388, -23.0505)
  point P4 (-34.0203, 0.0351)
  point P5 (-34.0203, 0.0351)
  point P6 (-26.7388, 21.5341)
  point P7 (-26.7388, 21.5341)
  dimension "d80" = 2.55
  dimension "d81" = 2.55
  dimension "d82" = 2.55
  dimension "d83" = 2.55
  dimension "d84" = 2.55
  constraint coincident P0 A0.centre
  constraint horizontal L12.end L14.end
  constraint coincident P1 A2.centre
  constraint horizontal L18.end L20.end
  constraint coincident P3 P2
  constraint horizontal L24.end L26.end
  constraint coincident P4 A4.centre
  constraint horizontal L30.end L32.end
  constraint coincident P7 P6
  constraint horizontal L36.end L38.end
  measures "d80" distance of P0 L15
  measures "d81" distance of P1 L21
  measures "d82" distance of L27 P3
  measures "d83" distance of L33 P5
  measures "d84" distance of L39 P7
extrude "Extrude3" cut sketch "Nut countersink" against normal blind 2.5 contours L10 L11 L12 L13 L14 L15 | L16 L17 L18 L19 L20 L21 | L22 L23 L24 L25 L26 L27 | L28 L29 L30 L31 L32 L33 | L34 L35 L36 L37 L38 L39 bodies 1 in component "Bottom frame"
sketch "Print helper membrane" plane through (0, 0, -1.5) normal (0, 0, -1) x (1, 0, 0) in component "Bottom frame"
  circle A0 centre (28.498, 0) radius 1.5
  line L0 (25.948, 1.4722) -> (25.948, -1.4722)
  line L1 (25.948, -1.4722) -> (28.498, -2.9445)
  line L2 (28.498, -2.9445) -> (31.048, -1.4722)
  line L3 (31.048, -1.4722) -> (31.048, 1.4722)
  line L4 (31.048, 1.4722) -> (28.498, 2.9445)
  line L5 (28.498, 2.9445) -> (25.948, 1.4722)
  circle A1 centre (28.498, 0) radius 1.5
  circle A2 centre (26.9591, 22.8364) radius 1.5
  circle A3 centre (-26.7388, 21.5341) radius 1.5
  circle A4 centre (-34.0203, 0.0351) radius 1.5
  circle A5 centre (-26.7388, -23.0505) radius 1.5
extrude "Extrude4" add sketch "Print helper membrane" against normal blind 0.1 contours A0 A1 | A2 | A3 | A4 | A5 bodies 1 in component "Bottom frame"
chamfer "Chamfer1" distance 0.75 angle 45 15 edges at (2.4201, 15.2167, -4) (31.8996, 2.1047, -4) (31.7195, -11.6871, -4) (29.6551, -25.7913, -4) (0.0131, -26.1841, -4) (-29.1091, -24.7562, -4) (-34.1681, -12.0677, -4) (-38.02, -0.0771, -4) (-34.1943, 12.7109, -4) (-28.4243, 26.678, -4) (0.037, 7.5426, -4) (-27.0263, 8.8414, -4) (-26.8295, -8.7969, -4) (-0.3107, -18.1739, -4) (23.7701, -10.6666, -4) on bodies 1 in component "Bottom frame"
chamfer "Chamfer2" distance 0.25 angle 45 30 edges at (25.948, 0, -4) (27.223, 2.2084, -4) (29.773, 2.2084, -4) (31.048, 0, -4) (29.773, -2.2084, -4) (27.223, -2.2084, -4) (28.2341, -20.628, -4) (25.6841, -20.628, -4) (24.4091, -22.8364, -4) (25.6841, -25.0447, -4) (28.2341, -25.0447, -4) (29.5091, -22.8364, -4) (-28.0138, 25.2589, -4) (-25.4638, 25.2589, -4) (-24.1888, 23.0505, -4) (-25.4638, 20.8421, -4) (-28.0138, 20.8421, -4) (-29.2888, 23.0505, -4) (-32.7453, 2.1733, -4) (-31.4703, -0.0351, -4) (-32.7453, -2.2434, -4) (-35.2953, -2.2434, -4) (-36.5703, -0.0351, -4) (-35.2953, 2.1733, -4) (-25.4638, -19.3258, -4) (-28.0138, -19.3258, -4) (-29.2888, -21.5341, -4) (-28.0138, -23.7425, -4) (-25.4638, -23.7425, -4) (-24.1888, -21.5341, -4) on bodies 1 in component "Bottom frame"
sketch "Top frame" plane through (0, 0, 0) normal (0, 0, 1) x (1, 0, 0) in component "Top frame"
  line L0 (23.6, -23.6) -> (-23.6, -23.6) construction
  line L1 (-23.6, -23.6) -> (-23.6, 23.6) construction
  line L2 (-23.6, 23.6) -> (23.6, 23.6) construction
  line L3 (23.6, 23.6) -> (23.6, -23.6) construction
  line L4 (-24.1, 24.1) -> (24.1, 24.1)
  line L5 (24.1, 24.1) -> (24.1, -24.1)
  line L6 (24.1, -24.1) -> (-24.1, -24.1)
  line L7 (-24.1, -24.1) -> (-24.1, 24.1)
  line L8 (0, 50) -> (0, -50) construction
  line L9 (-50, 0) -> (50, 0) construction
  circle A0 centre (-26.7388, 23.0505) radius 1.5
  circle A1 centre (-34.0203, -0.0351) radius 1.5
  circle A2 centre (-26.7388, -21.5341) radius 1.5
  circle A3 centre (26.9591, -22.8364) radius 1.5
  circle A4 centre (28.498, 0) radius 1.5
  circle A5 centre (-26.7388, -21.5341) radius 2.75
  circle A6 centre (-26.7388, -21.5341) radius 4 construction
  circle A7 centre (-34.0203, -0.0351) radius 2.75 construction
  circle A8 centre (-34.0203, -0.0351) radius 4 construction
  circle A9 centre (-26.7388, 23.0505) radius 2.75 construction
  circle A10 centre (-26.7388, 23.0505) radius 4 construction
  circle A11 centre (28.498, 0) radius 2.75 construction
  circle A12 centre (28.498, 0) radius 4 construction
  circle A13 centre (26.9591, -22.8364) radius 2.75 construction
  circle A14 centre (26.9591, -22.8364) radius 4 construction
  line L10 (3.7595, -26.7104) -> (-1.3205, -26.7104)
  line L11 (3.7595, -26.7104) -> (3.7595, -24.1)
  line L12 (-1.3205, -26.7104) -> (-1.3205, -24.1)
  line L13 (29.025, 29.1) -> (32.5142, 0.1054)
  line L14 (32.5142, 0.1054) -> (30.546, -29.1)
  line L15 (30.546, -29.1) -> (-28.3996, -29.1)
  line L16 (-28.3996, -29.1) -> (-38.2285, -0.0793)
  line L17 (-38.2285, -0.0793) -> (-29.025, 29.1)
  line L18 (-29.025, 29.1) -> (29.025, 29.1)
  point P0 (-26.7388, 23.0505)
  point P1 (-34.0203, -0.0351)
  point P2 (-26.7388, -21.5341)
  point P3 (26.9591, -22.8364)
  point P4 (28.498, 0)
  point P5 (2.4895, -25.4404)
  point P6 (-0.0505, -25.4404)
  dimension "d91" = 48.2
  dimension "d92" = 48.2
  dimension "d94" = 24.1
  dimension "d95" = 24.1
  dimension "d96" = 3
  dimension "d97" = 5.5
  dimension "d98" = 8
  dimension "d99" = 3
  dimension "d100" = 5.5
  dimension "d101" = 8
  dimension "d102" = 3
  dimension "d103" = 5.5
  dimension "d104" = 8
  dimension "d105" = 3
  dimension "d106" = 5.5
  dimension "d107" = 8
  dimension "d108" = 3
  dimension "d109" = 5.5
  dimension "d110" = 8
  dimension "d111" = 5.08
  dimension "d112" = 1.27
  dimension "d113" = 1.27
  dimension "d115" = 5
  dimension "d116" = 4.925
  dimension "d117" = 4.925
  dimension "d118" = 5
  constraint horizontal L4
  constraint vertical L5
  constraint horizontal L6
  constraint vertical L7
  constraint vertical L8
  constraint perpendicular L3 L9
  constraint coincident P0 A0.centre
  constraint coincident P1 A1.centre
  constraint coincident P2 A2.centre
  constraint coincident P3 A3.centre
  constraint coincident P4 A4.centre
  constraint concentric A5 A6
  constraint concentric A1 A7
  constraint concentric A7 A8
  constraint concentric A4 A11
  constraint concentric A3 A13
  constraint concentric A3 A14
  constraint perpendicular L8 L10
  constraint coincident L6 L11.end
  constraint perpendicular L6 L11
  constraint coincident L6 L12.end
  constraint perpendicular L6 L12
  constraint tangent A10 L17
  constraint tangent A8 L17
  constraint tangent A8 L16
  constraint tangent A6 L16
  constraint tangent A14 L14
  constraint tangent A12 L14
  constraint tangent A12 L13
  constraint horizontal L18
  measures "d91" distance of L4.start L4.end
  measures "d92" distance of L4.end L5.end
  measures "d94" distance of L5 L8
  measures "d95" distance of L4 L9
  measures "d96" diameter of A0
  measures "d97" diameter of A9
  measures "d98" diameter of A10
  measures "d99" diameter of A1
  measures "d100" diameter of A7
  measures "d101" diameter of A8
  measures "d102" diameter of A2
  measures "d103" diameter of A5
  measures "d104" diameter of A6
  measures "d105" diameter of A4
  measures "d106" diameter of A11
  measures "d107" diameter of A12
  measures "d108" diameter of A3
  measures "d109" diameter of A13
  measures "d110" diameter of A14
  measures "d111" distance of L10.start L10.end
  measures "d112" horizontal distance of P5 L10.start
  measures "d113" vertical distance of P6 L10.end
  measures "d115" distance of L6 L15
  measures "d116" horizontal distance of L4.start L17.end
  measures "d117" horizontal distance of L4.end L13.start
  measures "d118" distance of L4 L18
extrude "Extrude1'" add sketch "Top frame" along normal blind 8 separate body contours L7 A5 | L13 L14 L15 L16 L17 L18 picked at (-24.4796, -21.5341) makes body 6 in component "Top frame"
sketch "Skrew head countersink" plane through (0, 0, 8) normal (0, 0, 1) x (-1, 0, 0) in component "Top frame"
  circle A0 centre (26.7388, -23.0505) radius 1.5
  circle A1 centre (34.0203, 0.0351) radius 1.5
  circle A2 centre (-26.9591, 22.8364) radius 1.5
  line L0 (-3.7595, 24.1) -> (-3.7595, 26.7104)
  line L1 (-3.7595, 26.7104) -> (1.3205, 26.7104)
  line L2 (1.3205, 26.7104) -> (1.3205, 24.1)
  line L3 (1.3205, 24.1) -> (24.1, 24.1)
  line L4 (24.1, 24.1) -> (24.1, -24.1)
  line L5 (24.1, -24.1) -> (-24.1, -24.1)
  line L6 (-24.1, -24.1) -> (-24.1, 24.1)
  line L7 (-24.1, 24.1) -> (-3.7595, 24.1)
  circle A3 centre (26.7388, 21.5341) radius 1.5
  circle A4 centre (-28.498, 0) radius 1.5
  line L8 (29.025, -29.1) -> (38.2285, 0.0793)
  line L9 (38.2285, 0.0793) -> (28.3996, 29.1)
  line L10 (28.3996, 29.1) -> (-30.546, 29.1)
  line L11 (-30.546, 29.1) -> (-32.5142, -0.1054)
  line L12 (-32.5142, -0.1054) -> (-29.025, -29.1)
  line L13 (-29.025, -29.1) -> (29.025, -29.1)
  circle A5 centre (26.7388, 21.5341) radius 2.75
extrude "Extrude2'" cut sketch "Skrew head countersink" against normal blind 4 contours L4 A5 picked at (24.4796, 21.5341) bodies 6 in component "Top frame"
move_body "Move1" bodies 1 to x (1, 0, 0) y (0, 1, 0) z (0, 0, 1) at (0, 0, -2) in component "Bottom frame"
sketch "Heatsink locks" plane through (0, 0, 8) normal (0, 0, 1) x (-1, 0, 0) in component "Heatsink locks"
  line L0 (29.025, -29.1) -> (38.2285, 0.0793)
  line L1 (38.2285, 0.0793) -> (28.3996, 29.1)
  line L2 (28.3996, 29.1) -> (-30.546, 29.1)
  line L3 (-30.546, 29.1) -> (-32.5142, -0.1054)
  line L4 (-32.5142, -0.1054) -> (-29.025, -29.1)
  line L5 (-29.025, -29.1) -> (29.025, -29.1)
  circle A0 centre (-28.498, 0) radius 1.5
  arc A1 (24.1, 20.7601) -> (24.1, 22.3081) centre (26.7388, 21.5341) ccw
  line L6 (24.1, 20.7601) -> (24.1, -24.1)
  line L7 (24.1, -24.1) -> (-24.1, -24.1)
  line L8 (-24.1, -24.1) -> (-24.1, 24.1)
  line L9 (-24.1, 24.1) -> (-3.7595, 24.1)
  line L10 (-3.7595, 24.1) -> (-3.7595, 26.7104)
  line L11 (-3.7595, 26.7104) -> (1.3205, 26.7104)
  line L12 (1.3205, 26.7104) -> (1.3205, 24.1)
  line L13 (1.3205, 24.1) -> (24.1, 24.1)
  line L14 (24.1, 24.1) -> (24.1, 22.3081)
  circle A2 centre (-26.9591, 22.8364) radius 1.5
  circle A3 centre (34.0203, 0.0351) radius 1.5
  circle A4 centre (26.7388, -23.0505) radius 1.5
  line L15 (36.5619, 5) -> (24.1, 5)
  line L16 (24.1, -24.1) -> (24.1, -29.1)
  line L17 (24.1, -29.1) -> (29.025, -29.1)
  line L18 (38.2285, 0.0793) -> (29.025, -29.1)
  line L19 (38.2285, 0.0793) -> (36.5619, 5)
  line L20 (24.1, 5) -> (24.1, -24.1)
  line L21 (-31.9252, -5) -> (-24.1, -5)
  line L22 (-31.9252, -5) -> (-32.5142, -0.1054)
  line L23 (-30.546, 29.1) -> (-32.5142, -0.1054)
  line L24 (-24.1, -5) -> (-24.1, 29.1)
  line L25 (-24.1, 29.1) -> (-30.546, 29.1)
  circle A5 centre (26.7388, -23.0505) radius 1.5
  circle A6 centre (34.0203, 0.0351) radius 1.5
  circle A7 centre (-28.498, 0) radius 1.5
  circle A8 centre (-26.9591, 22.8364) radius 1.5
  point P0 (24.1, -8)
  point P1 (-24.1, 8)
  dimension "d123" = 5
  dimension "d124" = 5
  dimension "d125" = 8
  dimension "d126" = 8
  constraint coincident L1 L15.start
  constraint coincident L6 L15.end
  constraint perpendicular L6 L15
  constraint coincident L6.end L7.start
  constraint coincident L5 L16.end
  constraint perpendicular L5 L16
  constraint coincident L0.start L5.end
  constraint coincident L0.end L1.start
  constraint parallel L1 L19
  constraint perpendicular L7 L20
  constraint coincident L4 L21.start
  constraint coincident L8 L21.end
  constraint perpendicular L8 L21
  constraint coincident L3.end L4.start
  constraint coincident L2.end L3.start
  constraint coincident L2 L24.end
  constraint perpendicular L2 L24
  constraint coincident L20 P0
  constraint coincident L24 P1
  measures "d123" distance of origin L15
  measures "d124" vertical distance of origin L21.end
  measures "d125" vertical distance of origin P0
  measures "d126" vertical distance of origin P1
extrude "Extrude1''" add sketch "Heatsink locks" along normal blind 6 separate body contours L0 L1 L5 L6 L15 L16 L17 L18 L19 L20 | L2 L3 L4 L8 L21 L22 L23 L24 L25 makes body 7 at (-27.6906, 5.8214, 8) makes body 8 at (27.2391, -27.5107, 8) in component "Heatsink locks"